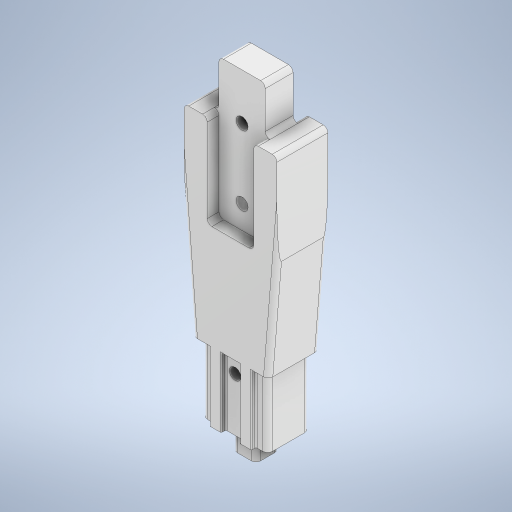
# Autodesk Inventor part: RP_Calf-Link
Saved by Autodesk Inventor 2024.3 (Build 283343000, 343)
## iProperties
Created: 2025-03-13
Part Number: RP_Calf-Link
Material: ABS プラスチック
Document SubType Name: Modeling
Designer: 佐藤智貴
Density: 1.06 g/cm^3
Appearance: 滑らか - 白
Mass: 82.2297 g
Surface Area: 167.621 cm^2
Volume: 77.5752 cm^3
Author: 佐藤智貴
Autodesk Inventor part; units mm, degrees
ref_plane "YZ Plane" through (0, 0, 0) normal (1, 0, 0) x (0, 1, 0)
ref_plane "XZ Plane" through (0, 0, 0) normal (0, 1, 0) x (-1, 0, 0)
ref_plane "XY Plane" through (0, 0, 0) normal (0, 0, 1) x (1, 0, 0)
sketch "スケッチ1" plane through (0, 0, 0) normal (0, 0, 1) x (1, 0, 0)
  line L0 (0, 0) -> (40, 0)
  line L1 (40, 0) -> (40, -120)
  line L2 (40, -120) -> (0, -120)
  line L3 (0, -120) -> (0, 0)
  line L4 (0, 0) -> (10, 0)
  line L5 (10, 0) -> (10, -50)
  line L6 (10, -50) -> (0, -50)
  line L7 (0, -50) -> (0, 0)
  line L8 (40, 0) -> (30, 0)
  line L9 (30, 0) -> (30, -50)
  line L10 (30, -50) -> (40, -50)
  line L11 (40, -50) -> (40, 0)
  line L12 (0, -10) -> (40, -10)
  line L13 (40, -10) -> (40, -50)
  line L14 (40, -50) -> (0, -50)
  line L15 (0, -50) -> (0, -10)
  circle A0 centre (20, -10) radius 2.6
  circle A1 centre (20, -40) radius 2.6
  line L16 (30, -50) -> (5, -50)
  line L17 (5, -120) -> (30, -120)
  line L18 (0, -120) -> (40, -120)
  line L19 (40, -120) -> (40, -110)
  line L20 (40, -110) -> (0, -110)
  line L21 (0, -110) -> (0, -120)
  line L22 (5, -50) -> (5, -120)
  line L23 (35, -50) -> (35, -120)
  line L24 (0, -50) -> (5, -110)
  line L25 (35, -110) -> (40, -50)
  line L26 (10, 0) -> (30, 0)
  line L27 (30, 0) -> (30, 10)
  line L28 (30, 10) -> (10, 10)
  line L29 (10, 10) -> (10, 0)
  point P0 (5, 0)
  point P1 (5, -50)
  point P2 (30, -10)
  point P3 (10, -10)
  point P4 (0, -50)
  point P5 (20, -50)
  point P6 (0, -50)
  dimension "d0" = 40
  dimension "d1" = 10
  dimension "d2" = 10
  dimension "d3" = 50
  dimension "d4" = 10
  dimension "d5" = 30
  dimension "d6" = 5.2
  dimension "d7" = 5.2
  dimension "d8" = 20
  dimension "d11" = 120
  dimension "d27" = 35
  dimension "d59" = 10
  dimension "d60" = 30
  dimension "d115" = 10
  dimension "d116" = 20
  constraints: 60 end point, 14 parallel, 10 point on line, 7 horizontal, 6 perpendicular, 4 midpoint, 2 centre point, 1 vertical
  measures "d0" distance between parallel lines of L3 L1
  measures "d1" distance between parallel lines of L3 L5
  measures "d2" distance between parallel lines of L1 L9
  measures "d3" distance of point (5, 0) point (5, -50)
  measures "d4" distance between parallel lines of L0 L12
  measures "d5" distance of A1.centre A0.centre
  measures "d6" diameter of A0
  measures "d7" diameter of A1
  measures "d8" distance from line of L13 A1.centre
  measures "d11" distance of L0.end L1.end
  measures "d27" distance of L2.end L23.end
  measures "d59" distance between parallel lines of L2 L20
  measures "d60" distance between parallel lines of L23 L22
  measures "d115" distance between parallel lines of L26 L28
  measures "d116" distance of L27.end L28.end
extrude "押し出し1" add sketch "スケッチ1" along normal blind 22 contours L29 L28 L27 L0 | L0 L9 L12 A0 L5 | L12 L5 L6 L3 | L12 A0 L9 L14 L5 | L6 L22 L24 | L12 L1 L10 L9 | L14 L10 L23 L20 L22 L6 | L20 L23 L2 L22 | L23 L10 L25
sketch "スケッチ2" plane through (0, 0, 22) normal (0, 0, 1) x (1, 0, 0)
  line L0 (10, 0) -> (30, 0)
  line L1 (30, 0) -> (30, -50)
  line L2 (30, -50) -> (10, -50)
  line L3 (10, -50) -> (10, 0)
  line L4 (30, -10) -> (30, 10) projected
  line L5 (10, 0) -> (30, 0)
  line L6 (30, 0) -> (30, 10)
  line L7 (30, 10) -> (10, 10)
  line L8 (10, 10) -> (10, 0)
  point P0 (0, 0)
  dimension "d12" = 20
  dimension "d13" = 50
  constraints: 16 end point, 4 parallel, 2 horizontal, 2 perpendicular
  measures "d12" distance between parallel lines of L3 L1
  measures "d13" distance of L0.end L1.end
extrude "押し出し2" cut sketch "スケッチ2" against normal blind 5
sketch "スケッチ3" plane through (0, 0, 0) normal (0, 0, -1) x (-1, 0, 0)
  line L0 (-30, -10) -> (-30, 10) projected
  line L1 (-30, 0) -> (-10, 0)
  line L2 (-10, 0) -> (-10, -50)
  line L3 (-10, -50) -> (-30, -50)
  line L4 (-30, -50) -> (-30, 0)
  line L5 (-10, 0) -> (-30, 0)
  line L6 (-30, 0) -> (-30, 10)
  line L7 (-30, 10) -> (-10, 10)
  line L8 (-10, 10) -> (-10, 0)
  point P0 (0, 0)
  point P1 (-20, -25)
  dimension "d19" = 20
  dimension "d20" = 50
  constraints: 16 end point, 4 parallel, 2 horizontal, 2 perpendicular
  measures "d19" distance between parallel lines of L4 L2
  measures "d20" distance of L1.end L2.end
extrude "押し出し3" cut sketch "スケッチ3" against normal blind 5
fillet "フィレット1" radius 2 14 edges at (30, -10, 19.5) (30, -10, 11) (30, -10, 2.5) (10, -10, 2.5) (10, -10, 11) (10, -10, 19.5) (0, -10, 11) (40, -10, 11) (30, -50, 2.5) (10, -50, 2.5) (10, -50, 19.5) (30, -50, 19.5) (30, 10, 11) (10, 10, 11)
sketch "スケッチ17" plane through (0, 0, 22) normal (0, 0, 1) x (1, 0, 0)
  line L0 (5, -110) -> (35, -110) projected
  line L1 (5, -110) -> (-34.5613, -110)
  line L2 (-34.5613, -110) -> (-34.5613, -152.4068)
  line L3 (-34.5613, -152.4068) -> (5, -152.4068)
  line L4 (5, -152.4068) -> (5, -110)
  line L5 (-34.5613, -110) -> (85.8131, -110)
  line L6 (85.8131, -110) -> (85.8131, -152.4068)
  line L7 (85.8131, -152.4068) -> (-34.5613, -152.4068)
  line L8 (-34.5613, -152.4068) -> (-34.5613, -110)
  point P0 (0, 0)
  constraints: 16 end point, 4 parallel, 2 horizontal, 2 perpendicular, 1 point on line
extrude "押し出し14" cut sketch "スケッチ17" along normal blind 30 and the other way blind 30
sketch "スケッチ18" plane through (5, -110, 22) normal (0, -1, 0) x (1, 0, 0)
  line L0 (30, -22) -> (0, -22) projected
  line L1 (30, -22) -> (30, 0) projected
  line L2 (0, 0) -> (30, 0) projected
  line L3 (0, -22) -> (0, 0) projected
  line L4 (0, -2) -> (30, -2)
  line L5 (30, -2) -> (30, -20)
  line L6 (30, -20) -> (0, -20)
  line L7 (0, -20) -> (0, -2)
  line L8 (1, -2) -> (29, -2)
  line L9 (29, -2) -> (29, -20)
  line L10 (29, -20) -> (1, -20)
  line L11 (1, -20) -> (1, -2)
  line L12 (0, 0) -> (30, 0)
  line L13 (30, 0) -> (30, -22)
  line L14 (30, -22) -> (0, -22)
  line L15 (0, -22) -> (0, 0)
  dimension "d123" = 30
  dimension "d124" = 18
  dimension "d125" = 2
  dimension "d126" = 1
  dimension "d127" = 1
  constraints: 24 end point, 6 parallel, 4 point on line, 3 horizontal, 3 perpendicular
  measures "d123" distance of L4.start L4.end
  measures "d124" distance between parallel lines of L6 L4
  measures "d125" distance between parallel lines of L2 L4
  measures "d126" distance between parallel lines of L3 L11
  measures "d127" distance between parallel lines of L1 L9
extrude "押し出し15" add sketch "スケッチ18" along normal blind 15
sketch "スケッチ19" plane through (5, -125, 22) normal (0, -1, 0) x (1, 0, 0)
  line L0 (10, -6) -> (20, -6)
  line L1 (20, -6) -> (20, -16)
  line L2 (20, -16) -> (10, -16)
  line L3 (10, -16) -> (10, -6)
  line L4 (28, -2) -> (2, -2) projected
  line L5 (30, -22) -> (30, 0) projected
  line L6 (28, -20) -> (28, -2) projected
  point P0 (-5, -22)
  point P1 (15, -6)
  dimension "d96" = 10
  dimension "d97" = 10
  dimension "d98" = 4
  dimension "d100" = 26
  dimension "d101" = 8
  constraints: 8 end point, 2 parallel, 1 horizontal, 1 midpoint, 1 perpendicular
  measures "d96" distance of L0.start L0.end
  measures "d97" distance of L0.end L1.end
  measures "d98" distance from line of L4 point (15, -6)
  measures "d100" distance of L4.start L4.end
  measures "d101" distance between parallel lines of L6 L1
extrude "押し出し16" add sketch "スケッチ19" along normal blind 10
sketch "スケッチ21" plane through (5, -110, 22) normal (0, -1, 0) x (1, 0, 0)
  line L0 (2, -2) -> (2, -20) projected
  line L1 (28, -20) -> (28, -2) projected
  line L2 (2, -2) -> (28, -2)
  line L3 (28, -2) -> (28, -20)
  line L4 (28, -20) -> (2, -20)
  line L5 (2, -20) -> (2, -2)
  line L6 (35, 5) -> (-5, 5)
  line L7 (-5, 5) -> (-5, -27)
  line L8 (-5, -27) -> (35, -27)
  line L9 (35, -27) -> (35, 5)
  line L10 (3, -22) -> (-3, -22) projected
  line L11 (33, 0) -> (27, 0) projected
  line L12 (0, -22) -> (30, -22)
  line L13 (30, -22) -> (30, 0)
  line L14 (30, 0) -> (0, 0)
  line L15 (0, 0) -> (0, -22)
  line L16 (2, -20) -> (28, -20)
  line L17 (28, -20) -> (28, -2)
  line L18 (28, -2) -> (2, -2)
  line L19 (2, -2) -> (2, -20)
  line L20 (1, -20) -> (29, -20)
  line L21 (29, -20) -> (29, -2)
  line L22 (29, -2) -> (1, -2)
  line L23 (1, -2) -> (1, -20)
  point P0 (-5, -22)
  dimension "d117" = 40
  dimension "d128" = 2
  dimension "d129" = 18
  dimension "d130" = 28
  dimension "d131" = 1
  constraints: 40 end point, 10 parallel, 5 perpendicular, 3 horizontal, 2 midpoint, 6 other
  measures "d117" distance of L6.start L6.end
  measures "d128" distance between parallel lines of L15 L19
  measures "d129" distance between parallel lines of L16 L18
  measures "d130" distance between parallel lines of L21 L23
  measures "d131" distance between parallel lines of L13 L21
extrude "押し出し18" cut sketch "スケッチ21" against normal blind 15 contours L9 L8 L7 L6 | L10 L15 L14 L11 L13 L12
sketch "スケッチ22" plane through (5, -125, 22) normal (0, -1, 0) x (1, 0, 0)
  line L0 (1, -20) -> (29, -20)
  line L1 (29, -20) -> (29, -2)
  line L2 (29, -2) -> (1, -2)
  line L3 (1, -2) -> (1, -20)
  line L4 (0, 0) -> (0, -22) projected
  line L5 (30, 0) -> (0, 0) projected
  line L6 (-5.5726, -27.0133) -> (33.6125, -27.0133)
  line L7 (33.6125, -27.0133) -> (33.6125, 10.2938)
  line L8 (33.6125, 10.2938) -> (-5.5726, 10.2938)
  line L9 (-5.5726, 10.2938) -> (-5.5726, -27.0133)
  point P0 (-5, -22)
  dimension "d132" = 28
  dimension "d133" = 1
  dimension "d134" = 18
  dimension "d135" = 2
  constraints: 16 end point, 4 parallel, 2 horizontal, 2 perpendicular
  measures "d132" distance between parallel lines of L1 L3
  measures "d133" distance between parallel lines of L4 L3
  measures "d134" distance between parallel lines of L0 L2
  measures "d135" distance between parallel lines of L5 L2
extrude "押し出し19" cut sketch "スケッチ22" against normal blind 15
fillet "フィレット5" radius 2 12 edges at (15, -130, 16) (15, -130, 6) (6, -110, 20) (6, -110, 2) (34, -110, 20) (34, -110, 2) (38.125, -72.5, 0) (38.125, -72.5, 22) (1.875, -72.5, 0) (1.875, -72.5, 22) (25, -130, 16) (25, -130, 6)
sketch "スケッチ23" plane through (32, -125, 2) normal (0, 0, -1) x (-1, 0, 0)
  circle A0 centre (12, 23) radius 2.5
  line L0 (-2.2431, 30) -> (26.2431, 30) projected
  line L1 (24, 30) -> (24, 0) projected
  point P0 (32, 125)
  dimension "d139" = 5
  dimension "d140" = 7
  dimension "d141" = 12
  constraints: 1 centre point
  measures "d139" diameter of A0
  measures "d140" distance from line of L0 A0.centre
  measures "d141" distance from line of L1 A0.centre
extrude "押し出し20" cut sketch "スケッチ23" against normal through all
sketch "スケッチ24" plane through (8, -95, 20) normal (0, 0, 1) x (1, 0, 0)
  line L0 (24, 0) -> (24, -30) projected
  line L1 (0, -30) -> (0, 0) projected
  line L2 (24, -30) -> (0, -30) projected
  line L3 (3, 0) -> (8, 0)
  line L4 (8, 0) -> (8, -30)
  line L5 (8, -30) -> (3, -30)
  line L6 (3, -30) -> (3, 0)
  line L7 (16, 0) -> (21, 0)
  line L8 (21, 0) -> (21, -30)
  line L9 (21, -30) -> (16, -30)
  line L10 (16, -30) -> (16, 0)
  point P0 (-8, 95)
  point P1 (16, -30)
  point P2 (3, -30)
  dimension "d147" = 24
  dimension "d153" = 5
  dimension "d154" = 5
  dimension "d155" = 3
  dimension "d156" = 3
  dimension "d157" = 30
  constraints: 16 end point, 4 parallel, 3 point on line, 2 horizontal, 2 perpendicular
  measures "d147" distance between parallel lines of L0 L1
  measures "d153" distance between parallel lines of L6 L4
  measures "d154" distance between parallel lines of L8 L10
  measures "d155" distance between parallel lines of L0 L8
  measures "d156" distance between parallel lines of L1 L6
  measures "d157" distance of L5.end L3.start
extrude "押し出し21" add sketch "スケッチ24" along normal blind 2 and the other way blind 20
fillet "フィレット6" radius 0.5 16 edges at (24, -110, 0) (24, -110, 2) (16, -110, 0) (11, -110, 0) (11, -110, 2) (29, -110, 0) (29, -110, 2) (16, -110, 2) (11, -110, 20) (11, -110, 22) (16, -110, 22) (24, -110, 20) (24, -110, 22) (16, -110, 20) (29, -110, 20) (29, -110, 22)
equation "\"d2\" = d1"
equation "\"d4\" = d2"
equation "\"d7\" = d6"
